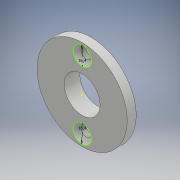
# Autodesk Inventor part: крышка
Saved by Autodesk Inventor 2018 (Build 220112000, 112)
## iProperties
Created: 2018-05-24
Part Number: крышка
Material: Типовые
Document SubType Name: Modeling
Designer: user
Density: 1 g/cm^3
Appearance: По умолчанию
Author: user
Autodesk Inventor part; units mm, degrees
ref_plane "YZ Plane" through (0, 0, 0) normal (1, 0, 0) x (0, 1, 0)
ref_plane "XZ Plane" through (0, 0, 0) normal (0, 1, 0) x (-1, 0, 0)
ref_plane "XY Plane" through (0, 0, 0) normal (0, 0, 1) x (1, 0, 0)
sketch "Эскиз1" plane through (0, 0, 0) normal (0, 1, 0) x (-1, 0, 0)
  point P0 (0, 0)
sketch "Эскиз2" plane through (0, 0, 0) normal (0, 1, 0) x (-1, 0, 0)
  circle A0 centre (0, 0) radius 40
  dimension "d0" = 80
  constraints: 1 centre point, 1 coincident
  measures "d0" diameter of A0
extrude "Выдавливание1" add sketch "Эскиз2" along normal blind 8
sketch "Эскиз3" plane through (0, 0, 0) normal (0, -1, 0) x (1, 0, 0)
  circle A0 centre (0, 30) radius 8.2
  circle A1 centre (0, -30) radius 8.2
  point P0 (0, 0)
  dimension "d3" = 16.4
  dimension "d4" = 16.4
  constraints: 2 centre point
  measures "d3" diameter of A0
  measures "d4" diameter of A1
sketch "Эскиз4" plane through (0, 0, 0) normal (1, 0, 0) x (0, 1, 0)
  line L0 (0, 40) -> (0, -40) projected
  line L1 (0, 29.8473) -> (0, 38.0473)
  line L2 (0, 38.0473) -> (8.2, 29.8473)
  line L3 (8.2, 29.8473) -> (0, 29.8473)
  point P0 (0, 0)
  dimension "d5" = 8.2
  dimension "d6" = 45
  constraints: 6 end point, 2 point on line, 1 perpendicular
  measures "d5" distance of L1.start L1.end
  measures "d6" angle of L1 L2
revolve "Вращение1" cut sketch "Эскиз4" angle 360 about axis through (0, 8.2, 29.8473) along (0, -1, 0)
sketch "Эскиз5" plane through (0, 0, 0) normal (1, 0, 0) x (0, 1, 0)
  point P0 (0, 0)
sketch "Эскиз6" plane through (0, 0, 0) normal (1, 0, 0) x (0, 1, 0)
  line L0 (0, 40) -> (0, -40) projected
  line L1 (0, -30) -> (0, -38.2)
  line L2 (0, -38.2) -> (8.2, -30)
  line L3 (8.2, -30) -> (0, -30)
  point P0 (0, 0)
  dimension "d8" = 8.2
  dimension "d9" = 45
  constraints: 6 end point, 2 point on line, 1 perpendicular
  measures "d8" distance of L1.start L1.end
  measures "d9" angle of L2 L1
revolve "Вращение2" cut sketch "Эскиз6" angle 360 about axis through (0, 8.2, -30) along (0, -1, 0)
sketch "Эскиз7" plane through (0, 8, 0) normal (0, 1, 0) x (1, 0, 0)
  circle A0 centre (0, 30) radius 0.2 projected
  circle A1 centre (0, -29.8473) radius 0.2 projected
  point P0 (0, 0)
  constraints: 2 coincident
hole "Отверстие1" at (0, 8, -30) at (0, 8, 29.8473) direction (0, -1, 0) diameter 9 end through all
sketch "Эскиз8" plane through (0, 8, 0) normal (0, 1, 0) x (1, 0, 0)
  circle A0 centre (0, 0) radius 22
  dimension "d18" = 44
  constraints: 1 centre point, 1 coincident
  measures "d18" diameter of A0
extrude "Выдавливание2" add sketch "Эскиз8" along normal blind 6
sketch "Эскиз9" plane through (0, 14, 0) normal (0, 1, 0) x (1, 0, 0)
  point P0 (0, 0)
  point P1 (0, 0)
  constraints: 1 coincident
hole "Отверстие2" at (0, 14, 0) direction (0, -1, 0) diameter 32 end through all
chamfer "Фаска1" distance 2 angle 45 1 edges at (-22, 14, 0)
